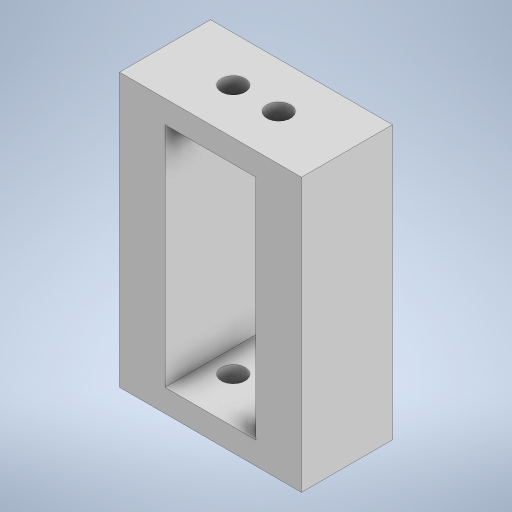
# Autodesk Inventor part: 다리 연결 부품
Saved by Autodesk Inventor 2024 (Build 280153000, 153)
## iProperties
Created: 2024-09-10
Part Number: 다리 연결 부품
Material: 일반
Document SubType Name: Modeling
Designer: USER
Density: 1 g/cm^3
Appearance: 기본값
Author: USER
Autodesk Inventor part; units mm, degrees
ref_plane "YZ Plane" through (0, 0, 0) normal (1, 0, 0) x (0, 1, 0)
ref_plane "XZ Plane" through (0, 0, 0) normal (0, 1, 0) x (-1, 0, 0)
sketch "스케치1" plane through (0, 0, 0) normal (0, 0, 1) x (1, 0, 0)
  line L0 (0, 0) -> (40, 0)
  line L1 (40, 0) -> (40, 60)
  line L2 (40, 60) -> (0, 60)
  line L3 (0, 60) -> (0, 0)
  line L4 (10, 5) -> (30, 5)
  line L5 (30, 5) -> (30, 55)
  line L6 (30, 55) -> (10, 55)
  line L7 (10, 55) -> (10, 5)
  point P0 (20, 55)
  point P1 (20, 60)
  point P2 (10, 30)
  point P3 (0, 30)
  dimension "d0" = 60
  dimension "d1" = 40
  dimension "d4" = 5
  dimension "d5" = 10
  constraints: 16 end point, 4 midpoint, 4 parallel, 2 horizontal, 2 perpendicular, 1 horizontal alignment, 1 vertical alignment
  measures "d0" distance of L0.end L1.end
  measures "d1" distance of L1.end L2.end
  measures "d4" distance between parallel lines of L2 L6
  measures "d5" distance between parallel lines of L3 L7
extrude "돌출1" add sketch "스케치1" along normal blind 20 contours L3 L2 L1 L0 | L7 L6 L5 L4
extrude "돌출2" cut sketch "스케치1" along normal blind 20 contours L7 L6 L5 L4
sketch "스케치2" plane through (0, 0, 0) normal (0, -1, 0) x (1, 0, 0)
  line L0 (10, 0) -> (10, 20) projected
  line L1 (0, 0) -> (40, 0) projected
  line L2 (40, 0) -> (40, 20) projected
  line L3 (0, 20) -> (40, 20) projected
  line L4 (0, 0) -> (0, 20) projected
  line L5 (30, 0) -> (30, 20) projected
  circle A0 centre (15, 10) radius 2.6
  circle A1 centre (25, 10) radius 2.6
  point P0 (10, 10)
  point P1 (20, 20)
  dimension "d11" = 5.2
  dimension "d12" = 5.2
  dimension "d13" = 10
  dimension "d14" = 5
  constraints: 2 centre point, 2 horizontal alignment, 2 midpoint
  measures "d11" diameter of A0
  measures "d12" diameter of A1
  measures "d13" distance of A1.centre A0.centre
  measures "d14" horizontal distance of A0.centre point (20, 20)
extrude "돌출3" cut sketch "스케치2" against normal through all contours A0 | A1
ref_plane "작업 평면1" through (0, 30, 0) normal (0, -1, 0) x (1, 0, 0)
